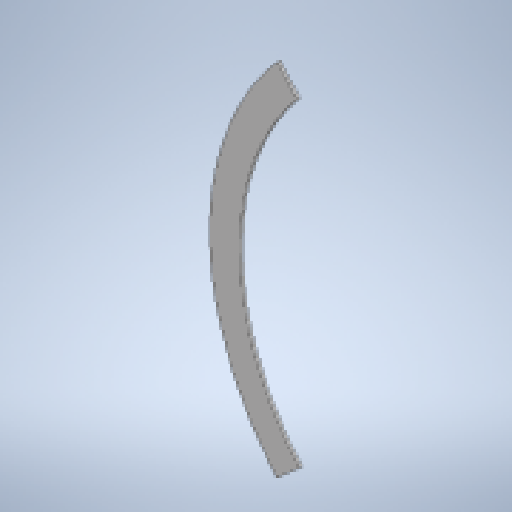
# Autodesk Inventor part: buzia
Saved by Autodesk Inventor 2023 (Build 270158000, 158)
## iProperties
Created: 2023-07-08
Part Number: buzia
Material: Ogólny
Document SubType Name: Modeling
Designer: Kamil
Density: 1 g/cm^3
Appearance: Domyślna
Author: Kamil
Autodesk Inventor part; units mm, degrees
ref_plane "YZ Plane" through (0, 0, 0) normal (1, 0, 0) x (0, 1, 0)
ref_plane "XZ Plane" through (0, 0, 0) normal (0, 1, 0) x (-1, 0, 0)
ref_plane "XY Plane" through (0, 0, 0) normal (0, 0, 1) x (1, 0, 0)
sketch "Szkic1" plane through (0, 0, 0) normal (0, 0, 1) x (1, 0, 0)
  arc A0 (-14.0761, 13.6183) -> (-14.1169, -13.5713) centre (1.5875, 0) ccw
  arc A1 (-12.5929, 11.902) -> (-12.4201, -12.1049) centre (1.5875, 0) ccw
  line L0 (-14.0761, 13.6183) -> (-12.5929, 11.902)
  line L1 (-12.4201, -12.1049) -> (-14.1169, -13.5713)
  point P0 (0, 0)
  constraints: 4 end point, 4 point on circle, 2 centre point, 1 perpendicular
extrude "Wyciągnięcie proste1" add sketch "Szkic1" along normal blind 0.2
